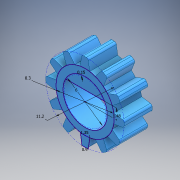
# Autodesk Inventor part: Motor Shaft Gear E
Saved by Autodesk Inventor 2018 (Build 220112000, 112)
## iProperties
Created: 2018-01-21
Part Number: Motor Shaft Gear E
Material: ABS Plastic
Document SubType Name: Modeling
Designer: Moochster
Density: 1.06 g/cm^3
Appearance: Smooth - White
Author: Moochster
Autodesk Inventor part; units mm, degrees
ref_plane "YZ Plane" through (0, 0, 0) normal (1, 0, 0) x (0, 1, 0)
ref_plane "XZ Plane" through (0, 0, 0) normal (0, 1, 0) x (-1, 0, 0)
ref_plane "XY Plane" through (0, 0, 0) normal (0, 0, 1) x (1, 0, 0)
sketch "Sketch1" plane through (0, 0, 0) normal (0, 1, 0) x (-1, 0, 0)
  arc A0 (0.45, -5.5819) -> (-0.45, -5.5819) centre (0, 0) ccw construction
  circle A1 centre (0, 0) radius 4.15
  line L0 (-0.45, -5.5819) -> (-0.675, -4.0947)
  line L1 (0.675, -4.0947) -> (0.45, -5.5819)
  line L2 (0.675, -4.0947) -> (-0.675, -4.0947) construction
  line L3 (0.45, -5.5819) -> (-0.45, -5.5819) construction
  arc A2 (-0.45, -5.5819) -> (0.45, -5.5819) centre (0, 0) ccw
  circle A3 centre (0, 0) radius 3 construction
  circle A4 centre (0, 0) radius 3.15
  line L4 (2.7807, 1.48) -> (-2.7807, 1.48)
  dimension "d1" = 11.2
  dimension "d2" = 8.3
  dimension "d3" = 0.9
  dimension "d4" = 1.35
  dimension "d13" = 6
  dimension "d16" = 0.15
  dimension "d17" = 1.48
  constraints: 10 end point, 8 point on circle, 5 centre point, 3 coincident, 3 horizontal, 1 equal length
  measures "d1" diameter of A0
  measures "d2" diameter of A1
  measures "d3" distance of L1.end L0.start
  measures "d4" distance of L1.start L0.end
  measures "d13" diameter of A3
  measures "d16" radial gap between concentric circles of A3 A4
  measures "d17" distance from line of A3.centre L4
extrude "Extrusion1" add sketch "Sketch1" along normal blind 4 contours A1 | A4 L4 | L4 A4
extrude "Extrusion2" add sketch "Sketch1" along normal blind 4 contours A1 L1 A2 L0
fillet "Fillet1" radius 0.3 2 edges at (0.45, 2, -5.5819) (-0.45, 2, -5.5819)
pattern_circular "Circular Pattern1" count 12 over 360 about axis through (0, 0, 0) along (0, 1, 0) of "Extrusion2", "Fillet1"
extrude "Extrusion3" cut sketch "Sketch1" along normal blind 4 contours A4 L4 picked at (1.2217, -1.3888)
body "Solid1"
